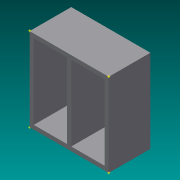
# Autodesk Inventor part: nano_enclosure_v3
Saved by Autodesk Inventor 2015 (Build 190159000, 159)
## iProperties
Created: 2015-03-02
Part Number: nano_enclosure_v3
Material: Generic
Document SubType Name: Modeling
Designer: Jeff
Density: 1 g/cm^3
Appearance: Default
Author: Jeff
Autodesk Inventor part; units mm, degrees
ref_plane "YZ Plane" through (0, 0, 0) normal (1, 0, 0) x (0, 1, 0)
ref_plane "XZ Plane" through (0, 0, 0) normal (0, 1, 0) x (-1, 0, 0)
ref_plane "XY Plane" through (0, 0, 0) normal (0, 0, 1) x (1, 0, 0)
sketch "Sketch2" plane through (0, 0, 0) normal (0, 0, 1) x (1, 0, 0)
  line L0 (0, 0) -> (48.26, 0)
  line L1 (48.26, 0) -> (48.26, 50.8)
  line L2 (48.26, 50.8) -> (0, 50.8)
  line L3 (0, 50.8) -> (0, 0)
  dimension "d0" = 50.8
  dimension "d1" = 48.26
  constraints: 8 end point, 2 parallel, 1 horizontal, 1 perpendicular
  measures "d0" distance of L0.end L1.end
  measures "d1" distance of L1.end L2.end
extrude "Extrusion1" add sketch "Sketch2" along normal blind 25.4
sketch "Sketch3" plane through (0, 0, 25.4) normal (0, 0, 1) x (1, 0, 0)
  line L0 (2.54, 2.54) -> (22.86, 2.54)
  line L1 (22.86, 2.54) -> (22.86, 48.26)
  line L2 (22.86, 48.26) -> (2.54, 48.26)
  line L3 (2.54, 48.26) -> (2.54, 2.54)
  line L4 (0, 0) -> (48.26, 0) projected
  line L5 (0, 50.8) -> (0, 0) projected
  line L6 (48.26, 50.8) -> (0, 50.8) projected
  line L7 (25.4, 2.54) -> (45.72, 2.54)
  line L8 (45.72, 2.54) -> (45.72, 48.26)
  line L9 (45.72, 48.26) -> (25.4, 48.26)
  line L10 (25.4, 48.26) -> (25.4, 2.54)
  line L11 (48.26, 0) -> (48.26, 50.8) projected
  dimension "d4" = 2.54
  dimension "d5" = 2.54
  dimension "d6" = 2.54
  dimension "d7" = 22.86
  dimension "d8" = 2.54
  dimension "d9" = 2.54
  dimension "d10" = 2.54
  dimension "d11" = 22.86
  constraints: 16 end point, 4 parallel, 2 horizontal, 2 perpendicular
  measures "d4" distance between parallel lines of L4 L0
  measures "d5" distance between parallel lines of L5 L3
  measures "d6" distance between parallel lines of L6 L2
  measures "d7" distance between parallel lines of L5 L1
  measures "d8" distance between parallel lines of L4 L7
  measures "d9" distance between parallel lines of L11 L8
  measures "d10" distance between parallel lines of L6 L9
  measures "d11" distance between parallel lines of L11 L10
extrude "Extrusion2" cut sketch "Sketch3" against normal blind 20.32 contours L3 L2 L1 L0 | L10 L9 L8 L7
sketch "Sketch4" plane through (0, 0, 0) normal (0, 0, -1) x (-1, 0, 0)
  circle A0 centre (-12.7, 19.05) radius 8.89
  line L0 (0, 50.8) -> (0, 0) projected
  line L1 (0, 0) -> (-48.26, 0) projected
  dimension "d14" = 17.78
  dimension "d17" = 12.7
  dimension "d18" = 19.05
  constraints: 1 centre point
  measures "d14" diameter of A0
  measures "d17" distance from line of L0 A0.centre
  measures "d18" distance from line of L1 A0.centre
extrude "Extrusion3" cut sketch "Sketch4" against normal blind 2.54
sketch "Sketch5" plane through (0, 0, 0) normal (0, 0, -1) x (-1, 0, 0)
  point P0 (0, 0)
sketch "Sketch6" plane through (12.7, 19.05, 2.54) normal (0, 0, -1) x (-1, 0, 0)
  circle A0 centre (0, 0) radius 8.89 projected
  line L0 (0, 0) -> (-5.08, 0)
  line L1 (-5.08, 0) -> (-5.08, 19.05)
  line L2 (-5.08, 19.05) -> (0, 19.05)
  line L3 (0, 19.05) -> (0, 0)
  line L4 (0, 0) -> (5.08, 0)
  line L5 (5.08, 0) -> (5.08, 19.05)
  line L6 (5.08, 19.05) -> (0, 19.05)
  line L7 (0, 19.05) -> (0, 0)
  point P0 (12.7, -19.05)
  dimension "d21" = 19.05
  dimension "d22" = 5.08
  dimension "d23" = 5.08
  constraints: 16 end point, 4 parallel, 2 horizontal, 2 perpendicular, 1 point on line
  measures "d21" distance between parallel lines of L4 L6
  measures "d22" distance of L0.start L0.end
  measures "d23" distance between parallel lines of L3 L5
extrude "Extrusion4" cut sketch "Sketch6" along normal blind 2.54 contours L5 L4 L3 A0 | A0 L3 L6 L5 | L1 L2 L3 A0 | A0 L3 L0 L1
sketch "Sketch7" plane through (0, 0, 2.54) normal (0, 0, -1) x (-1, 0, 0)
  point P0 (0, 0)
sketch "Sketch8" plane through (0, 0, 2.54) normal (0, 0, -1) x (-1, 0, 0)
  line L0 (-7.62, 26.3456) -> (-7.62, 38.1) projected
  line L1 (-17.78, 38.1) -> (-7.62, 38.1)
  line L2 (-7.62, 38.1) -> (-7.62, 34.29)
  line L3 (-7.62, 34.29) -> (-17.78, 34.29)
  line L4 (-17.78, 34.29) -> (-17.78, 38.1)
  point P0 (0, 0)
  dimension "d26" = 3.81
  constraints: 8 end point, 2 parallel, 1 horizontal, 1 perpendicular, 1 point on line
  measures "d26" distance between parallel lines of L1 L3
extrude "Extrusion5" cut sketch "Sketch8" against normal blind 2.54
sketch "Sketch9" plane through (0, 0, 5.08) normal (0, 0, 1) x (1, 0, 0)
  line L0 (43.815, 45.1783) -> (27.94, 45.1783)
  line L1 (27.94, 45.1783) -> (27.94, 26.1283)
  line L2 (27.94, 26.1283) -> (43.815, 26.1283)
  line L3 (43.815, 26.1283) -> (43.815, 45.1783)
  line L4 (25.4, 2.54) -> (25.4, 48.26) projected
  point P0 (0, 0)
  dimension "d29" = 26.1283
  dimension "d30" = 2.54
  dimension "d31" = 15.875
  dimension "d32" = 19.05
  constraints: 8 end point, 2 parallel, 1 horizontal, 1 perpendicular
  measures "d29" distance from line of L2 point (0, 0)
  measures "d30" distance between parallel lines of L1 L4
  measures "d31" distance between parallel lines of L3 L1
  measures "d32" distance between parallel lines of L2 L0
extrude "Extrusion6" cut sketch "Sketch9" against normal blind 1.27
sketch "Sketch10" plane through (0, 0, 3.81) normal (0, 0, 1) x (1, 0, 0)
  line L0 (27.94, 45.1783) -> (43.815, 45.1783) projected
  line L1 (32.7025, 45.1783) -> (39.0525, 45.1783)
  line L2 (39.0525, 45.1783) -> (39.0525, 37.5583)
  line L3 (39.0525, 37.5583) -> (32.7025, 37.5583)
  line L4 (32.7025, 37.5583) -> (32.7025, 45.1783)
  line L5 (43.815, 45.1783) -> (43.815, 26.1283) projected
  line L6 (27.94, 26.1283) -> (27.94, 45.1783) projected
  point P0 (0, 0)
  dimension "d35" = 6.35
  dimension "d36" = 7.62
  dimension "d37" = 4.7625
  dimension "d38" = 4.7625
  constraints: 8 end point, 2 parallel, 1 horizontal, 1 perpendicular, 1 point on line
  measures "d35" distance between parallel lines of L2 L4
  measures "d36" distance between parallel lines of L3 L0
  measures "d37" distance between parallel lines of L5 L2
  measures "d38" distance between parallel lines of L6 L4
extrude "Extrusion7" cut sketch "Sketch10" against normal blind 3.81
body "Solid1"
